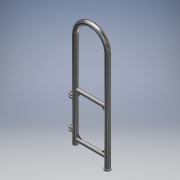
# Autodesk Inventor part: Door Frame
Saved by Autodesk Inventor 2018 (Build 220112000, 112)
## iProperties
Created: 2018-02-10
Part Number: Door Frame
Material: Steel, Alloy
Document SubType Name: Modeling
Designer: Joey
Density: 7.73 g/cm^3
Appearance: Semi-Polished
Author: Joey
Autodesk Inventor part; units mm, degrees
ref_plane "XZ Plane" through (0, 0, 0) normal (0, 1, 0) x (-1, 0, 0)
ref_plane "XY Plane" through (0, 0, 0) normal (0, 0, 1) x (1, 0, 0)
sketch "Sketch1" plane through (0, 0, 0) normal (0, 1, 0) x (-1, 0, 0)
  circle A0 centre (-171.45, 0) radius 25.4
  circle A1 centre (171.45, 0) radius 25.4
  line L0 (171.45, 0) -> (-171.45, 0) construction
  point P0 (0, 0)
  point P1 (0, 0)
  dimension "d0" = 50.8
  dimension "d1" = 50.8
  dimension "d2" = 342.9
  constraints: 2 centre point, 2 end point, 1 coincident, 1 horizontal, 1 midpoint
  measures "d0" diameter of A0
  measures "d1" diameter of A1
  measures "d2" distance of L0.end L0.start
extrude "Extrusion1" add sketch "Sketch1" along normal blind 1016
sketch "Sketch2" plane through (0, 0, 0) normal (0, 0, 1) x (1, 0, 0)
  line L0 (-146.05, 1016) -> (-196.85, 1016) projected
  line L1 (196.85, 1016) -> (146.05, 1016) projected
  arc A0 (171.45, 1016) -> (-171.45, 1016) centre (0, 1016) ccw
  point P0 (0, 0)
  constraints: 2 midpoint, 2 point on circle, 1 centre point, 1 point on line
sketch "Sketch3" plane through (171.45, 1016, 0) normal (0, 1, 0) x (1, 0, 0)
  circle A0 centre (0, 0) radius 25.4 projected
  circle A1 centre (-342.9, 0) radius 25.4 projected
  point P0 (-171.45, 0)
sweep "Sweep1" add profiles "Sketch3" path "Sketch2" path curves A0 contours A0
ref_plane "Work Plane1" through (-171.45, 0, 0) normal (1, 0, 0) x (0, 1, 0)
sketch "Sketch4" plane through (-171.45, 0, 0) normal (1, 0, 0) x (0, 1, 0)
  circle A0 centre (508, 0) radius 19.05
  line L0 (0, 25.4) -> (0, -25.4) projected
  circle A1 centre (50.8, 0) radius 19.05
  point P0 (0, 0)
  dimension "d8" = 38.1
  dimension "d9" = 508
  dimension "d10" = 38.1
  dimension "d11" = 50.8
  constraints: 2 centre point
  measures "d8" diameter of A0
  measures "d9" distance from line of A0.centre L0
  measures "d10" diameter of A1
  measures "d11" distance from line of A1.centre L0
extrude "Extrusion2" add sketch "Sketch4" along normal up to next
sketch "Sketch5" plane through (-171.45, 0, 0) normal (1, 0, 0) x (0, 1, 0)
  line L0 (0, 25.4) -> (1016, 25.4) construction
  line L1 (457.2, -25.4) -> (444.5, -25.4)
  line L2 (444.5, -25.4) -> (444.5, 25.4)
  line L3 (444.5, 25.4) -> (457.2, 25.4)
  line L4 (457.2, 25.4) -> (457.2, -25.4)
  line L5 (431.8, -25.4) -> (419.1, -25.4)
  line L6 (419.1, -25.4) -> (419.1, 25.4)
  line L7 (419.1, 25.4) -> (431.8, 25.4)
  line L8 (431.8, 25.4) -> (431.8, -25.4)
  line L9 (0, -25.4) -> (1016, -25.4) construction
  arc A0 (508, -19.05) -> (508, -19.05) centre (508, 0) ccw construction
  line L10 (1016, -25.4) -> (1016, 25.4) construction
  line L11 (0, 25.4) -> (0, -25.4) construction
  line L12 (114.3, -25.4) -> (127, -25.4)
  line L13 (127, -25.4) -> (127, 25.4)
  line L14 (127, 25.4) -> (114.3, 25.4)
  line L15 (114.3, 25.4) -> (114.3, -25.4)
  line L16 (139.7, -25.4) -> (152.4, -25.4)
  line L17 (152.4, -25.4) -> (152.4, 25.4)
  line L18 (152.4, 25.4) -> (139.7, 25.4)
  line L19 (139.7, 25.4) -> (139.7, -25.4)
  spline S0 degree 3 poles (508, -19.05) (506.7208, -19.05) (505.4369, -18.9199) (502.9363, -18.409) (501.7189, -18.0285) (499.4082, -17.0487) (498.3125, -16.4485) (496.2868, -15.0732) (495.3568, -14.2976) (493.7198, -12.6606) (492.948, -11.7406) (491.5679, -9.7155) (490.9596, -8.6102) (489.9684, -6.2749) (489.5848, -5.0422) (489.0755, -2.531) (488.95, -1.2523) (488.95, 1.2523) (489.0755, 2.531) (489.5848, 5.0422) (489.9684, 6.2749) (490.9596, 8.6102) (491.5679, 9.7155) (492.948, 11.7406) (493.7198, 12.6606) (495.3568, 14.2976) (496.2868, 15.0732) (498.3125, 16.4485) (499.4082, 17.0487) (501.7189, 18.0285) (502.9363, 18.409) (505.4369, 18.9199) (506.7208, 19.05) (509.2792, 19.05) (510.5631, 18.9199) (513.0637, 18.409) (514.2811, 18.0285) (516.5918, 17.0487) (517.6875, 16.4485) (519.7132, 15.0732) (520.6432, 14.2976) (522.2802, 12.6606) (523.052, 11.7406) (524.4321, 9.7155) (525.0404, 8.6102) (526.0316, 6.2749) (526.4152, 5.0422) (526.9245, 2.531) (527.05, 1.2523) (527.05, -1.2523) (526.9245, -2.531) (526.4152, -5.0422) (526.0316, -6.2749) (525.0404, -8.6102) (524.4321, -9.7155) (523.052, -11.7406) (522.2802, -12.6606) (520.6432, -14.2976) (519.7132, -15.0732) (517.6875, -16.4485) (516.5918, -17.0487) (514.2811, -18.0285) (513.0637, -18.409) (510.5631, -18.9199) (509.2792, -19.05) (508, -19.05) knots 0 0 0 0 0.383756 0.383756 0.767512 0.767512 1.151268 1.151268 1.535024 1.535024 1.910709 1.910709 2.286393 2.286393 2.662078 2.662078 3.037763 3.037763 3.413447 3.413447 3.789132 3.789132 4.164816 4.164816 4.540501 4.540501 4.924257 4.924257 5.308013 5.308013 5.691769 5.691769 6.075525 6.075525 6.459281 6.459281 6.843037 6.843037 7.226793 7.226793 7.61055 7.61055 7.986234 7.986234 8.361919 8.361919 8.737603 8.737603 9.113288 9.113288 9.488972 9.488972 9.864657 9.864657 10.240341 10.240341 10.616026 10.616026 10.999782 10.999782 11.383538 11.383538 11.767294 11.767294 12.15105 12.15105 12.15105 12.15105 construction
  spline S1 degree 3 poles (50.8, -19.05) (49.5208, -19.05) (48.2369, -18.9199) (45.7363, -18.409) (44.5189, -18.0285) (42.2082, -17.0487) (41.1125, -16.4485) (39.0868, -15.0732) (38.1568, -14.2976) (36.5198, -12.6606) (35.748, -11.7406) (34.3679, -9.7155) (33.7596, -8.6102) (32.7684, -6.2749) (32.3848, -5.0422) (31.8755, -2.531) (31.75, -1.2523) (31.75, 1.2523) (31.8755, 2.531) (32.3848, 5.0422) (32.7684, 6.2749) (33.7596, 8.6102) (34.3679, 9.7155) (35.748, 11.7406) (36.5198, 12.6606) (38.1568, 14.2976) (39.0868, 15.0732) (41.1125, 16.4485) (42.2082, 17.0487) (44.5189, 18.0285) (45.7363, 18.409) (48.2369, 18.9199) (49.5208, 19.05) (52.0792, 19.05) (53.3631, 18.9199) (55.8637, 18.409) (57.0811, 18.0285) (59.3918, 17.0487) (60.4875, 16.4485) (62.5132, 15.0732) (63.4432, 14.2976) (65.0802, 12.6606) (65.852, 11.7406) (67.2321, 9.7155) (67.8404, 8.6102) (68.8316, 6.2749) (69.2152, 5.0422) (69.7245, 2.531) (69.85, 1.2523) (69.85, -1.2523) (69.7245, -2.531) (69.2152, -5.0422) (68.8316, -6.2749) (67.8404, -8.6102) (67.2321, -9.7155) (65.852, -11.7406) (65.0802, -12.6606) (63.4432, -14.2976) (62.5132, -15.0732) (60.4875, -16.4485) (59.3918, -17.0487) (57.0811, -18.0285) (55.8637, -18.409) (53.3631, -18.9199) (52.0792, -19.05) (50.8, -19.05) knots 0 0 0 0 0.383756 0.383756 0.767512 0.767512 1.151268 1.151268 1.535024 1.535024 1.910709 1.910709 2.286393 2.286393 2.662078 2.662078 3.037763 3.037763 3.413447 3.413447 3.789132 3.789132 4.164816 4.164816 4.540501 4.540501 4.924257 4.924257 5.308013 5.308013 5.691769 5.691769 6.075525 6.075525 6.459281 6.459281 6.843037 6.843037 7.226793 7.226793 7.61055 7.61055 7.986234 7.986234 8.361919 8.361919 8.737603 8.737603 9.113288 9.113288 9.488972 9.488972 9.864657 9.864657 10.240341 10.240341 10.616026 10.616026 10.999782 10.999782 11.383538 11.383538 11.767294 11.767294 12.15105 12.15105 12.15105 12.15105 construction
  line L20 (1016, -25.4) -> (1016, 25.4) construction
  line L21 (0, 25.4) -> (0, -25.4) construction
  point P0 (0, 0)
  point P1 (1016, 25.4)
  point P2 (1016, -25.4)
  dimension "d15" = 12.7
  dimension "d16" = 12.7
  dimension "d17" = 12.7
  dimension "d18" = 12.7
  dimension "d19" = 12.7
  dimension "d20" = 12.7
  dimension "d26" = 50.8
  dimension "d88" = 114.3
  constraints: 32 end point, 8 parallel, 5 horizontal, 4 perpendicular, 2 point on circle, 1 centre point, 1 point on line, 12 other
  measures "d15" distance between parallel lines of L2 L4
  measures "d16" distance between parallel lines of L6 L8
  measures "d17" distance between parallel lines of L8 L2
  measures "d18" distance between parallel lines of L19 L17
  measures "d19" distance between parallel lines of L13 L19
  measures "d20" distance between parallel lines of L15 L13
  measures "d26" distance from line of L4 A0.centre
  measures "d88" distance from line of point (0, 0) L15
extrude "Extrusion3" add sketch "Sketch5" against normal blind 63.5
fillet "Fillet1" radius 25.4 8 edges at (-234.95, 450.85, 25.4) (-234.95, 450.85, -25.4) (-234.95, 425.45, -25.4) (-234.95, 425.45, 25.4) (-234.95, 146.05, 25.4) (-234.95, 146.05, -25.4) (-234.95, 120.65, -25.4) (-234.95, 120.65, 25.4)
sketch "Sketch6" plane through (-171.45, 457.2, 0) normal (0, 1, 0) x (1, 0, 0)
  line L0 (0, 25.4) -> (-63.5, 25.4) projected
  line L1 (0, 35.56) -> (0, -35.56) projected
  point P0 (171.45, 0)
  point P1 (-44.45, 0)
  point P2 (-38.1, 25.4)
  point P3 (88.9, 25.4)
  dimension "d27" = 25.4
  dimension "d28" = 44.45
  constraints: 1 other
  measures "d27" distance from line of L0 point (-44.45, 0)
hole "Hole1" at (-215.9, 457.2, 0) direction (0, -1, 0) diameter 19.05 end through all
sketch "Sketch7" plane through (0, 0, 0) normal (0, 0, 1) x (1, 0, 0)
  line L0 (-146.05, 488.95) -> (146.05, 488.95) construction
  line L1 (-146.05, 0) -> (-146.05, 1016) construction
  line L2 (146.05, 0) -> (146.05, 1016) construction
  line L3 (-146.05, 69.85) -> (146.05, 69.85) construction
  line L4 (146.05, 488.95) -> (107.95, 488.95) construction
  line L5 (146.05, 488.95) -> (146.05, 450.85) construction
  line L6 (-146.05, 488.95) -> (-107.95, 488.95) construction
  line L7 (-146.05, 488.95) -> (-146.05, 450.85) construction
  line L8 (-146.05, 450.85) -> (-107.95, 488.95)
  line L9 (-158.75, 501.65) -> (-158.75, 438.15)
  line L10 (-158.75, 438.15) -> (-146.05, 450.85)
  line L11 (-107.95, 488.95) -> (-95.25, 501.65)
  line L12 (-95.25, 501.65) -> (-158.75, 501.65)
  line L13 (-146.05, 488.95) -> (146.05, 488.95) projected
  line L14 (0, 488.95) -> (0, 69.85) construction
  line L15 (0, 279.4) -> (-146.05, 279.4) construction
  line L16 (-146.05, 69.85) -> (-107.95, 69.85) construction
  line L17 (-146.05, 69.85) -> (-146.05, 107.95) construction
  line L18 (-146.05, 107.95) -> (-107.95, 69.85)
  line L19 (-158.75, 57.15) -> (-158.75, 120.65)
  line L20 (-158.75, 120.65) -> (-146.05, 107.95)
  line L21 (-107.95, 69.85) -> (-95.25, 57.15)
  line L22 (-95.25, 57.15) -> (-158.75, 57.15)
  line L23 (146.05, 488.95) -> (107.95, 488.95) construction
  line L24 (146.05, 488.95) -> (146.05, 450.85) construction
  line L25 (146.05, 450.85) -> (107.95, 488.95)
  line L26 (158.75, 501.65) -> (158.75, 438.15)
  line L27 (158.75, 438.15) -> (146.05, 450.85)
  line L28 (107.95, 488.95) -> (95.25, 501.65)
  line L29 (95.25, 501.65) -> (158.75, 501.65)
  line L30 (146.05, 69.85) -> (107.95, 69.85) construction
  line L31 (107.95, 69.85) -> (95.25, 57.15)
  line L32 (95.25, 57.15) -> (158.75, 57.15)
  line L33 (146.05, 107.95) -> (107.95, 69.85)
  line L34 (146.05, 69.85) -> (146.05, 107.95) construction
  line L35 (158.75, 57.15) -> (158.75, 120.65)
  line L36 (158.75, 120.65) -> (146.05, 107.95)
  point P0 (0, 0)
  point P1 (146.05, 279.4)
  dimension "d39" = 38.1
  dimension "d83" = 12.7
  dimension "d84" = 38.1
  dimension "d85" = 12.7
  constraints: 64 end point, 21 symmetric about line, 9 point on line, 3 midpoint, 2 collinear, 1 horizontal, 1 perpendicular, 1 vertical
  measures "d39" distance of L0.start L7.end
  measures "d83" distance between parallel lines of L0 L12
  measures "d84" distance of L0.start L6.end
  measures "d85" distance between parallel lines of L1 L9
extrude "Extrusion4" add sketch "Sketch7" along normal mid plane 6.35
sketch "Sketch8" plane through (171.45, 0, 0) normal (0, -1, 0) x (1, 0, 0)
  circle A0 centre (0, 0) radius 25.4 projected
  point P0 (-171.45, 0)
extrude "Extrusion5" add sketch "Sketch8" along normal blind 63.5
sketch "Sketch9" plane through (171.45, -63.5, 0) normal (0, -1, 0) x (1, 0, 0)
  circle A0 centre (0, 0) radius 25.4 construction
  circle A1 centre (0, 0) radius 31.75
  point P0 (-171.45, 0)
  dimension "d56" = 63.5
  constraints: 1 centre point, 1 coincident
  measures "d56" diameter of A1
extrude "Extrusion6" add sketch "Sketch9" against normal blind 12.7
sketch "Sketch11" plane through (0, 0, 3.175) normal (0, 0, 1) x (1, 0, 0)
  line L0 (-107.6836, 489.2164) -> (-146.2492, 489.2164) construction
  line L1 (-107.6836, 489.2164) -> (-146.2492, 450.6508) construction
  line L2 (146.2492, 450.6508) -> (107.6836, 489.2164) construction
  line L3 (146.2492, 489.2164) -> (107.6836, 489.2164) construction
  line L4 (146.2492, 450.6508) -> (146.2492, 489.2164) construction
  line L5 (-146.2492, 489.2164) -> (-146.2492, 450.6508) construction
  line L6 (146.2492, 69.5836) -> (146.2492, 108.1492) construction
  line L7 (107.6836, 69.5836) -> (146.2492, 69.5836) construction
  line L8 (107.6836, 69.5836) -> (146.2492, 108.1492) construction
  line L9 (-146.2492, 108.1492) -> (-146.2492, 69.5836) construction
  line L10 (-146.2492, 108.1492) -> (-107.6836, 69.5836) construction
  line L11 (-146.2492, 69.5836) -> (-107.6836, 69.5836) construction
  line L12 (-107.95, 488.95) -> (107.95, 488.95) construction
  line L13 (-107.95, 69.85) -> (107.95, 69.85) construction
  line L14 (0, 488.95) -> (0, 69.85) construction
  line L15 (0, 279.4) -> (90.999, 279.4) construction
  point P0 (0, 0)
  point P1 (-133.5492, 476.5164)
  point P2 (133.5492, 476.5164)
  point P3 (-133.5492, 82.2836)
  point P4 (133.5492, 82.2836)
  dimension "d86" = 12.7
  dimension "d87" = 12.7
  constraints: 4 end point, 3 midpoint, 3 symmetric about line, 1 horizontal
  measures "d86" distance from line of point (-133.549, 476.516) L0
  measures "d87" distance from line of L5 point (-133.549, 476.516)
hole "Hole2" at (-133.5492, 476.5164, 3.175) at (133.5492, 476.5164, 3.175) at (133.5492, 82.2836, 3.175) at (-133.5492, 82.2836, 3.175) direction (0, 0, -1) diameter 10.5918 end through all
body "Solid1"
